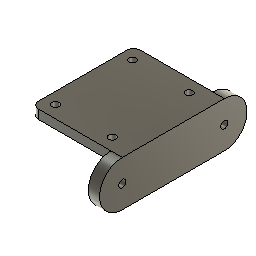
D415 Camera Mount (Autodesk Fusion 360 design; units mm, degrees)
Autodesk Fusion 360 part; units mm, degrees
sketch "Sketch1" plane through (0, 0, 0) normal (0, 0, 1) x (1, 0, 0)
  line L0 (0, 0) -> (0, 45)
  circle A0 centre (0, 0) radius 1.6
  circle A1 centre (0, 45) radius 1.6
  line L1 (10, 0) -> (10, 45)
  arc A2 (10, 45) -> (-10, 45) centre (0, 45) ccw
  line L2 (-10, 45) -> (-10, 0)
  arc A3 (-10, 0) -> (10, 0) centre (0, 0) ccw
  line L3 (0, 0) -> (0, 45) construction
  dimension "d1" = 45
  dimension "d2" = 3.2
  dimension "d3" = 3.2
  dimension "d4" = 20
  constraint coincident L0.start A0.centre
  constraint vertical L0
  constraint coincident L0.end A1.centre
  constraint tangent L1 A2
  constraint tangent A2 L2
  constraint parallel L1 L2
  constraint tangent L2 A3
  constraint tangent L1 A3
  constraint parallel L0 L3
  measures "d1" distance of L0.start L0.end
  measures "d2" diameter of A0
  measures "d3" diameter of A1
  measures "d4" diameter of A2
extrude "Extrude1" add sketch "Sketch1" along normal blind 5
sketch "Sketch2" plane through (0, 0, 0) normal (0, 0, -1) x (1, 0, 0)
  circle A0 centre (0, -45) radius 1.6
  circle A1 centre (0, 0) radius 1.6
  arc A2 (10, 0) -> (-10, 0) centre (0, 0) ccw
  line L0 (-10, 0) -> (-10, -45)
  arc A3 (-10, -45) -> (10, -45) centre (0, -45) ccw
  line L1 (10, -45) -> (10, 0)
  line L2 (10, 0) -> (6, 0)
  line L3 (6, 0) -> (6, -45)
  line L4 (6, -45) -> (10, -45)
  line L5 (10, -45) -> (10, 0)
  dimension "d7" = 4
  dimension "d8" = 45
  constraint horizontal L2
  constraint vertical L3
  constraint horizontal L4
  constraint vertical L5
  constraint coincident A2.start L1.end
  measures "d7" distance of A2.start L2.end
  measures "d8" distance of A2.start A3.end
extrude "Extrude2" add sketch "Sketch2" along normal blind 35 contours L1 L2 L3 L4 L5
fillet "Fillet1" radius 3 2 edges at (8, 0, -35) (8, 45, -35)
sketch "Sketch3" plane through (10, 0, 0) normal (1, 0, 0) x (0, 1, 0)
  arc A0 (42, -35) -> (45, -32) centre (42, -32) ccw
  line L0 (45, -32) -> (45, 0)
  line L1 (45, 0) -> (45, 5)
  line L2 (45, 5) -> (0, 5)
  line L3 (0, 5) -> (0, 0)
  line L4 (0, 0) -> (0, -32)
  arc A1 (0, -32) -> (3, -35) centre (3, -32) ccw
  line L5 (3, -35) -> (42, -35)
  line L6 (22.5, 5) -> (22.5, -35)
  line L7 (22.5, 5) -> (39.5, 5) construction
  line L8 (39.5, 5) -> (39.5, -35) construction
  line L9 (39.5, 5) -> (39.5, -5) construction
  circle A2 centre (39.5, -5) radius 1.6
  line L10 (39.5, -5) -> (39.5, -30) construction
  circle A3 centre (39.5, -30) radius 1.6
  circle A4 centre (5.5, -5) radius 1.6
  circle A5 centre (5.5, -30) radius 1.6
  dimension "d13" = 17
  dimension "d14" = 3.2
  dimension "d15" = 25
  dimension "d16" = 3.2
  constraint midpoint L2 L6.start
  constraint midpoint L5 L6.end
  constraint perpendicular L6 L7
  constraint coincident L5 L8.end
  constraint perpendicular L5 L8
  constraint coincident L8 L9.end
  constraint coincident L9.end A2.centre
  constraint coincident L8 L10.end
  constraint coincident L10.end A3.centre
  constraint symmetric L6 A2 A4
  constraint symmetric L6 A3 A5
  measures "d13" distance of L6.start L7.end
  measures "d14" diameter of A2
  measures "d15" distance of L9.end L10.end
  measures "d16" diameter of A3
extrude "Extrude3" cut sketch "Sketch3" against normal blind 16 contours A2 | A3 | A4 | A5
ref_plane "WorkPlane1" through (8, 33, -17.5) normal (0, 1, 0) x (1, 0, 0)
sketch "Sketch4" plane through (7.5, 33, -16) normal (0, 1, 0) x (1, 0, 0)
  line L0 (-17.5, -16) -> (2.5, -16)
  line L1 (2.5, -16) -> (2.5, -21)
  line L2 (-17.5, -21) -> (2.5, -21)
  line L3 (-17.5, -21) -> (-17.5, -16)
  line L4 (-1.5, 16) -> (2.5, 16)
  line L5 (2.5, 16) -> (2.5, -16)
  line L6 (2.5, -16) -> (-1.5, -16)
  line L7 (-1.5, -16) -> (-1.5, 16)
  line L8 (-7.5, -21) -> (-7.5, -16)
  line L9 (-7.5, -21) -> (-17.5, -21) construction
  line L10 (-12.5, -21) -> (-12.5, -16)
  line L11 (-12.5, -16) -> (-1.5, -5)
  line L12 (-12.5, -16) -> (1.6421, -16) construction
  dimension "d20" = 45
  constraint midpoint L2 L8.start
  constraint midpoint L0 L8.end
  constraint coincident L2.start L3.start
  constraint midpoint L9 L10.start
  constraint coincident L0 L10.end
  constraint perpendicular L0 L10
  constraint horizontal L12
  constraint coincident L7 L11.end
  measures "d20" angle of L11 L12
extrude "Extrude4" add sketch "Sketch4" against normal blind 5 contours L0 L7 L11
ref_plane "WorkPlane2" through (8, 22.5, -17.5) normal (0, 1, 0) x (1, 0, 0)
mirror "Mirror1" about plane through (8, 22.5, -17.5) normal (0, 1, 0) of "Extrude4"
move_body "Move1" bodies 1 to x (0, 0, -1) y (0, 1, 0) z (1, 0, 0) at (25, 0, -5)
move_body "Move2" bodies 1 to x (1, 0, 0) y (0, -1, 0) z (0, 0, -1) at (0, 52.2279, -22)
